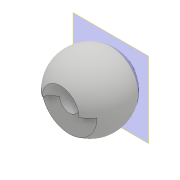
# Autodesk Inventor part: sensor_pad
Saved by Autodesk Inventor 2017 (Build 210142000, 142)
## iProperties
Created: 2018-05-30
Part Number: sensor_pad
Material: Generic
Document SubType Name: Modeling
Designer: Nic
Density: 1 g/cm^3
Appearance: Default
Author: Nic
Autodesk Inventor part; units mm, degrees
ref_plane "YZ Plane" through (0, 0, 0) normal (1, 0, 0) x (0, 1, 0)
ref_plane "XY Plane" through (0, 0, 0) normal (0, 0, 1) x (1, 0, 0)
sketch "Sketch1" plane through (0, 0, 0) normal (0, 0, 1) x (1, 0, 0)
  arc A0 (0, -15) -> (0, 15) centre (0, 0) ccw
  line L0 (0, 15) -> (0, -15)
  dimension "d0" = 30
  constraints: 2 end point, 2 point on circle, 1 centre point, 1 coincident, 1 midpoint, 1 vertical
  measures "d0" diameter of A0
revolve "Revolution1" add sketch "Sketch1" angle 360 about axis through (0, 15, 0) along (0, -1, 0)
sketch "Sketch2" plane through (0, 0, 0) normal (0, 0, 1) x (1, 0, 0)
  arc A0 (-9, 17) -> (9, 17) centre (0, 17) ccw
  line L0 (-9, 17) -> (9, 17)
  point P0 (0, 0)
  dimension "d2" = 17
  dimension "d13" = 9
  dimension "d19" = 18
  constraints: 2 end point, 2 point on circle, 1 centre point, 1 horizontal, 1 midpoint, 1 vertical alignment
  measures "d2" distance of point (0, 0) A0.centre
  measures "d13" radius of A0
  measures "d19" distance of L0.start L0.end
revolve "Revolution2" cut sketch "Sketch2" angle 360 about axis through (-9, 17, 0) along (1, 0, 0)
mirror "Mirror1" about plane through (0, 0, 0) normal (0, 1, 0) of "Revolution2"
ref_plane "Work Plane1" through (0, 9, 0) normal (0, 1, 0) x (-1, 0, 0)
sketch "Sketch3" plane through (0, 9, 0) normal (0, 1, 0) x (-1, 0, 0)
  line L0 (0, 0) -> (19, 0)
  line L1 (19, 0) -> (19, -16)
  line L2 (19, -16) -> (-19, -16)
  line L3 (-19, -16) -> (-19, 0)
  line L4 (-19, 0) -> (0, 0)
  line L5 (0, 0) -> (0, -16) construction
  dimension "d15" = 38
  dimension "d16" = 16
  constraints: 12 end point, 1 collinear, 1 horizontal, 1 midpoint, 1 parallel, 1 perpendicular, 1 point on line, 1 vertical, 1 other
  measures "d15" distance of L1.end L2.end
  measures "d16" distance of L2.end L3.end
extrude "Extrusion1" cut sketch "Sketch3" along normal blind 10
mirror "Mirror2" about plane through (0, 0, 0) normal (0, 1, 0) of "Extrusion1"
body "Solid1"
